Autodesk Fusion 360 part; units mm, degrees
note: some values were not read from the file. Set by a fixed rule: which face or edge a step refers to.
(part 7 of 13)
sketch "Sketch1 (3)" plane through (0, 0, 5) normal (0, 0, 1) x (-1, 0, 0)
  arc A0 (-3.482098, 1.419763) -> (-3.725467, 0.511498) centre (0, 0) ccw
  line L0 (-3.725467, 0.511498) -> (-4.55596, 0.625523)
  line L1 (-4.55596, 0.625523) -> (-4.55639, 0.625578)
  spline S0 degree 5 poles (-4.55639, 0.625578) (-4.556439, 0.625584) (-4.556519, 0.625594) (-4.556664, 0.625612) (-4.556887, 0.625638) (-4.557214, 0.625675) (-4.557589, 0.625717) (-4.558012, 0.625763) (-4.558483, 0.625812) (-4.559001, 0.625865) (-4.559566, 0.625921) (-4.560177, 0.62598) (-4.560835, 0.62604) (-4.561539, 0.626103) (-4.562289, 0.626167) (-4.563084, 0.626233) (-4.563925, 0.626299) (-4.564811, 0.626366) (-4.565742, 0.626434) (-4.566718, 0.626502) (-4.567738, 0.62657) (-4.568802, 0.626637) (-4.569909, 0.626704) (-4.571061, 0.626769) (-4.572255, 0.626834) (-4.573493, 0.626896) (-4.574774, 0.626957) (-4.576097, 0.627016) (-4.577463, 0.627072) (-4.578871, 0.627126) (-4.580321, 0.627176) (-4.581812, 0.627224) (-4.583345, 0.627268) (-4.584919, 0.627308) (-4.586534, 0.627345) (-4.58819, 0.627377) (-4.589886, 0.627405) (-4.591623, 0.627428) (-4.5934, 0.627446) (-4.595217, 0.627459) (-4.597073, 0.627467) (-4.598968, 0.627469) (-4.600903, 0.627465) (-4.602877, 0.627456) (-4.60489, 0.627439) (-4.606941, 0.627417) (-4.60903, 0.627387) (-4.611158, 0.627351) (-4.613323, 0.627308) (-4.615527, 0.627257) (-4.617767, 0.627198) (-4.620045, 0.627132) (-4.62236, 0.627058) (-4.624712, 0.626975) (-4.6271, 0.626884) (-4.629525, 0.626785) (-4.631986, 0.626676) (-4.634484, 0.626559) (-4.637017, 0.626432) (-4.639585, 0.626296) (-4.642189, 0.626151) (-4.644828, 0.625996) (-4.647503, 0.62583) (-4.650212, 0.625655) (-4.652956, 0.625469) (-4.655734, 0.625273) (-4.658546, 0.625066) (-4.661393, 0.624848) (-4.664273, 0.624619) (-4.667187, 0.624379) (-4.670135, 0.624128) (-4.673116, 0.623865) (-4.67613, 0.62359) (-4.679177, 0.623304) (-4.682256, 0.623005) (-4.685368, 0.622694) (-4.688513, 0.622371) (-4.691689, 0.622035) (-4.694898, 0.621687) (-4.698138, 0.621325) (-4.70141, 0.620951) (-4.704714, 0.620563) (-4.708048, 0.620163) (-4.711414, 0.619748) (-4.714811, 0.61932) (-4.718238, 0.618879) (-4.721696, 0.618423) (-4.725184, 0.617953) (-4.728702, 0.61747) (-4.732251, 0.616971) (-4.735829, 0.616459) (-4.739437, 0.615931) (-4.743074, 0.615389) (-4.74674, 0.614832) (-4.750436, 0.61426) (-4.754161, 0.613673) (-4.757914, 0.613071) (-4.761696, 0.612453) (-4.765506, 0.611819) (-4.769345, 0.61117) (-4.773212, 0.610505) (-4.777106, 0.609824) (-4.781029, 0.609127) (-4.784979, 0.608414) (-4.788956, 0.607684) (-4.792961, 0.606938) (-4.796992, 0.606176) (-4.801051, 0.605396) (-4.805136, 0.6046) (-4.809248, 0.603787) (-4.813386, 0.602957) (-4.817551, 0.60211) (-4.821742, 0.601246) (-4.825958, 0.600364) (-4.830201, 0.599464) (-4.834469, 0.598547) (-4.838762, 0.597613) (-4.843081, 0.59666) (-4.847425, 0.59569) (-4.851793, 0.594701) (-4.856187, 0.593695) (-4.860605, 0.59267) (-4.865048, 0.591627) (-4.869515, 0.590565) (-4.874006, 0.589485) (-4.878521, 0.588386) (-4.88306, 0.587269) (-4.887623, 0.586132) (-4.892209, 0.584977) (-4.896819, 0.583802) (-4.901452, 0.582609) (-4.906108, 0.581396) (-4.910787, 0.580163) (-4.915489, 0.578912) (-4.920213, 0.577641) (-4.92496, 0.57635) (-4.929729, 0.57504) (-4.93452, 0.573709) (-4.939334, 0.572359) (-4.944169, 0.570989) (-4.949026, 0.569599) (-4.953904, 0.568189) (-4.958804, 0.566758) (-4.963725, 0.565307) (-4.968668, 0.563836) (-4.973631, 0.562344) (-4.978615, 0.560832) (-4.98362, 0.559299) (-4.988645, 0.557746) (-4.993691, 0.556171) (-4.998756, 0.554576) (-5.003842, 0.55296) (-5.008948, 0.551323) (-5.014074, 0.549664) (-5.01922, 0.547985) (-5.024384, 0.546284) (-5.029569, 0.544562) (-5.034772, 0.542818) (-5.039995, 0.541053) (-5.045236, 0.539267) (-5.050497, 0.537458) (-5.055776, 0.535628) (-5.061073, 0.533777) (-5.066389, 0.531903) (-5.071723, 0.530008) (-5.077076, 0.528091) (-5.082446, 0.526151) (-5.087834, 0.52419) (-5.093239, 0.522206) (-5.098663, 0.5202) (-5.104103, 0.518172) (-5.109561, 0.516122) (-5.115036, 0.514049) (-5.120528, 0.511953) (-5.126037, 0.509835) (-5.131563, 0.507695) (-5.137105, 0.505532) (-5.142663, 0.503346) (-5.148238, 0.501137) (-5.153829, 0.498906) (-5.159436, 0.496651) (-5.165059, 0.494374) (-5.170698, 0.492073) (-5.176352, 0.48975) (-5.182022, 0.487404) (-5.187708, 0.485034) (-5.193408, 0.482641) (-5.199124, 0.480225) (-5.204854, 0.477785) (-5.210599, 0.475322) (-5.21636, 0.472836) (-5.222134, 0.470326) (-5.227923, 0.467793) (-5.233727, 0.465236) (-5.239544, 0.462655) (-5.245376, 0.460051) (-5.251221, 0.457423) (-5.257081, 0.454771) (-5.262954, 0.452096) (-5.26884, 0.449396) (-5.27474, 0.446673) (-5.280653, 0.443925) (-5.28658, 0.441154) (-5.292519, 0.438359) (-5.298471, 0.435539) (-5.304436, 0.432696) (-5.310414, 0.429828) (-5.316404, 0.426936) (-5.322407, 0.42402) (-5.328422, 0.421079) (-5.334448, 0.418115) (-5.340487, 0.415125) (-5.346538, 0.412112) (-5.352601, 0.409074) (-5.358675, 0.406011) (-5.364761, 0.402924) (-5.370858, 0.399812) (-5.376966, 0.396676) (-5.383086, 0.393515) (-5.389216, 0.39033) (-5.395357, 0.387119) (-5.40151, 0.383884) (-5.407672, 0.380625) (-5.413846, 0.37734) (-5.420029, 0.374031) (-5.426223, 0.370696) (-5.432428, 0.367337) (-5.438642, 0.363953) (-5.444866, 0.360544) (-5.4511, 0.35711) (-5.457343, 0.353651) (-5.463597, 0.350166) (-5.469859, 0.346657) (-5.476131, 0.343123) (-5.482412, 0.339563) (-5.488702, 0.335979) (-5.495001, 0.332369) (-5.501309, 0.328733) (-5.507626, 0.325073) (-5.513951, 0.321387) (-5.520284, 0.317676) (-5.525358, 0.314687) (-5.529167, 0.312434) (-5.531709, 0.310927) (-5.53298, 0.310172) knots 0 0 0 0 0 0 0.00416667 0.00833333 0.0125 0.01666667 0.02083333 0.025 0.02916667 0.03333333 0.0375 0.04166667 0.04583333 0.05 0.05416667 0.05833333 0.0625 0.06666667 0.07083333 0.075 0.07916667 0.08333333 0.0875 0.09166667 0.09583333 0.1 0.10416667 0.10833333 0.1125 0.11666667 0.12083333 0.125 0.12916667 0.13333333 0.1375 0.14166667 0.14583333 0.15 0.15416667 0.15833333 0.1625 0.16666667 0.17083333 0.175 0.17916667 0.18333333 0.1875 0.19166667 0.19583333 0.2 0.20416667 0.20833333 0.2125 0.21666667 0.22083333 0.225 0.22916667 0.23333333 0.2375 0.24166667 0.24583333 0.25 0.25416667 0.25833333 0.2625 0.26666667 0.27083333 0.275 0.27916667 0.28333333 0.2875 0.29166667 0.29583333 0.3 0.30416667 0.30833333 0.3125 0.31666667 0.32083333 0.325 0.32916667 0.33333333 0.3375 0.34166667 0.34583333 0.35 0.35416667 0.35833333 0.3625 0.36666667 0.37083333 0.375 0.37916667 0.38333333 0.3875 0.39166667 0.39583333 0.4 0.40416667 0.40833333 0.4125 0.41666667 0.42083333 0.425 0.42916667 0.43333333 0.4375 0.44166667 0.44583333 0.45 0.45416667 0.45833333 0.4625 0.46666667 0.47083333 0.475 0.47916667 0.48333333 0.4875 0.49166667 0.49583333 0.5 0.50416667 0.50833333 0.5125 0.51666667 0.52083333 0.525 0.52916667 0.53333333 0.5375 0.54166667 0.54583333 0.55 0.55416667 0.55833333 0.5625 0.56666667 0.57083333 0.575 0.57916667 0.58333333 0.5875 0.59166667 0.59583333 0.6 0.60416667 0.60833333 0.6125 0.61666667 0.62083333 0.625 0.62916667 0.63333333 0.6375 0.64166667 0.64583333 0.65 0.65416667 0.65833333 0.6625 0.66666667 0.67083333 0.675 0.67916667 0.68333333 0.6875 0.69166667 0.69583333 0.7 0.70416667 0.70833333 0.7125 0.71666667 0.72083333 0.725 0.72916667 0.73333333 0.7375 0.74166667 0.74583333 0.75 0.75416667 0.75833333 0.7625 0.76666667 0.77083333 0.775 0.77916667 0.78333333 0.7875 0.79166667 0.79583333 0.8 0.80416667 0.80833333 0.8125 0.81666667 0.82083333 0.825 0.82916667 0.83333333 0.8375 0.84166667 0.84583333 0.85 0.85416667 0.85833333 0.8625 0.86666667 0.87083333 0.875 0.87916667 0.88333333 0.8875 0.89166667 0.89583333 0.9 0.90416667 0.90833333 0.9125 0.91666667 0.92083333 0.925 0.92916667 0.93333333 0.9375 0.94166667 0.94583333 0.95 0.95416667 0.95833333 0.9625 0.96666667 0.97083333 0.975 0.97916667 0.98333333 0.9875 0.99166667 0.99583333 1 1 1 1 1 1
  arc A1 (-5.53298, 0.310172) -> (-5.53298, -0.310172) centre (0, 0) ccw
  spline S1 degree 5 poles (-5.53298, -0.310172) (-5.531709, -0.310927) (-5.529167, -0.312434) (-5.525358, -0.314687) (-5.520284, -0.317676) (-5.513951, -0.321387) (-5.507626, -0.325073) (-5.501309, -0.328733) (-5.495001, -0.332369) (-5.488702, -0.335979) (-5.482412, -0.339563) (-5.476131, -0.343123) (-5.469859, -0.346657) (-5.463597, -0.350166) (-5.457343, -0.353651) (-5.4511, -0.35711) (-5.444866, -0.360544) (-5.438642, -0.363953) (-5.432428, -0.367337) (-5.426223, -0.370696) (-5.420029, -0.374031) (-5.413846, -0.37734) (-5.407672, -0.380625) (-5.40151, -0.383884) (-5.395357, -0.387119) (-5.389216, -0.39033) (-5.383086, -0.393515) (-5.376966, -0.396676) (-5.370858, -0.399812) (-5.364761, -0.402924) (-5.358675, -0.406011) (-5.352601, -0.409074) (-5.346538, -0.412112) (-5.340487, -0.415125) (-5.334448, -0.418115) (-5.328422, -0.421079) (-5.322407, -0.42402) (-5.316404, -0.426936) (-5.310414, -0.429828) (-5.304436, -0.432696) (-5.298471, -0.435539) (-5.292519, -0.438359) (-5.28658, -0.441154) (-5.280653, -0.443925) (-5.27474, -0.446673) (-5.26884, -0.449396) (-5.262954, -0.452096) (-5.257081, -0.454771) (-5.251221, -0.457423) (-5.245376, -0.460051) (-5.239544, -0.462655) (-5.233727, -0.465236) (-5.227923, -0.467793) (-5.222134, -0.470326) (-5.21636, -0.472836) (-5.210599, -0.475322) (-5.204854, -0.477785) (-5.199124, -0.480225) (-5.193408, -0.482641) (-5.187708, -0.485034) (-5.182022, -0.487404) (-5.176352, -0.48975) (-5.170698, -0.492073) (-5.165059, -0.494374) (-5.159436, -0.496651) (-5.153829, -0.498906) (-5.148238, -0.501137) (-5.142663, -0.503346) (-5.137105, -0.505532) (-5.131563, -0.507695) (-5.126037, -0.509835) (-5.120528, -0.511953) (-5.115036, -0.514049) (-5.109561, -0.516122) (-5.104103, -0.518172) (-5.098663, -0.5202) (-5.093239, -0.522206) (-5.087834, -0.52419) (-5.082446, -0.526151) (-5.077076, -0.528091) (-5.071723, -0.530008) (-5.066389, -0.531903) (-5.061073, -0.533777) (-5.055776, -0.535628) (-5.050497, -0.537458) (-5.045236, -0.539267) (-5.039995, -0.541053) (-5.034772, -0.542818) (-5.029569, -0.544562) (-5.024384, -0.546284) (-5.01922, -0.547985) (-5.014074, -0.549664) (-5.008948, -0.551323) (-5.003842, -0.55296) (-4.998756, -0.554576) (-4.993691, -0.556171) (-4.988645, -0.557746) (-4.98362, -0.559299) (-4.978615, -0.560832) (-4.973631, -0.562344) (-4.968668, -0.563836) (-4.963725, -0.565307) (-4.958804, -0.566758) (-4.953904, -0.568189) (-4.949026, -0.569599) (-4.944169, -0.570989) (-4.939334, -0.572359) (-4.93452, -0.573709) (-4.929729, -0.57504) (-4.92496, -0.57635) (-4.920213, -0.577641) (-4.915489, -0.578912) (-4.910787, -0.580163) (-4.906108, -0.581396) (-4.901452, -0.582609) (-4.896819, -0.583802) (-4.892209, -0.584977) (-4.887623, -0.586132) (-4.88306, -0.587269) (-4.878521, -0.588386) (-4.874006, -0.589485) (-4.869515, -0.590565) (-4.865048, -0.591627) (-4.860605, -0.59267) (-4.856187, -0.593695) (-4.851793, -0.594701) (-4.847425, -0.59569) (-4.843081, -0.59666) (-4.838762, -0.597613) (-4.834469, -0.598547) (-4.830201, -0.599464) (-4.825958, -0.600364) (-4.821742, -0.601246) (-4.817551, -0.60211) (-4.813386, -0.602957) (-4.809248, -0.603787) (-4.805136, -0.6046) (-4.801051, -0.605396) (-4.796992, -0.606176) (-4.792961, -0.606938) (-4.788956, -0.607684) (-4.784979, -0.608414) (-4.781029, -0.609127) (-4.777106, -0.609824) (-4.773212, -0.610505) (-4.769345, -0.61117) (-4.765506, -0.611819) (-4.761696, -0.612453) (-4.757914, -0.613071) (-4.754161, -0.613673) (-4.750436, -0.61426) (-4.74674, -0.614832) (-4.743074, -0.615389) (-4.739437, -0.615931) (-4.735829, -0.616459) (-4.732251, -0.616971) (-4.728702, -0.61747) (-4.725184, -0.617953) (-4.721696, -0.618423) (-4.718238, -0.618879) (-4.714811, -0.61932) (-4.711414, -0.619748) (-4.708048, -0.620163) (-4.704714, -0.620563) (-4.70141, -0.620951) (-4.698138, -0.621325) (-4.694898, -0.621687) (-4.691689, -0.622035) (-4.688513, -0.622371) (-4.685368, -0.622694) (-4.682256, -0.623005) (-4.679177, -0.623304) (-4.67613, -0.62359) (-4.673116, -0.623865) (-4.670135, -0.624128) (-4.667187, -0.624379) (-4.664273, -0.624619) (-4.661393, -0.624848) (-4.658546, -0.625066) (-4.655734, -0.625273) (-4.652956, -0.625469) (-4.650212, -0.625655) (-4.647503, -0.62583) (-4.644828, -0.625996) (-4.642189, -0.626151) (-4.639585, -0.626296) (-4.637017, -0.626432) (-4.634484, -0.626559) (-4.631986, -0.626676) (-4.629525, -0.626785) (-4.6271, -0.626884) (-4.624712, -0.626975) (-4.62236, -0.627058) (-4.620045, -0.627132) (-4.617767, -0.627198) (-4.615527, -0.627257) (-4.613323, -0.627308) (-4.611158, -0.627351) (-4.60903, -0.627387) (-4.606941, -0.627417) (-4.60489, -0.627439) (-4.602877, -0.627456) (-4.600903, -0.627465) (-4.598968, -0.627469) (-4.597073, -0.627467) (-4.595217, -0.627459) (-4.5934, -0.627446) (-4.591623, -0.627428) (-4.589886, -0.627405) (-4.58819, -0.627377) (-4.586534, -0.627345) (-4.584919, -0.627308) (-4.583345, -0.627268) (-4.581812, -0.627224) (-4.580321, -0.627176) (-4.578871, -0.627126) (-4.577463, -0.627072) (-4.576097, -0.627016) (-4.574774, -0.626957) (-4.573493, -0.626896) (-4.572255, -0.626834) (-4.571061, -0.626769) (-4.569909, -0.626704) (-4.568802, -0.626637) (-4.567738, -0.62657) (-4.566718, -0.626502) (-4.565742, -0.626434) (-4.564811, -0.626366) (-4.563925, -0.626299) (-4.563084, -0.626233) (-4.562289, -0.626167) (-4.561539, -0.626103) (-4.560835, -0.62604) (-4.560177, -0.62598) (-4.559566, -0.625921) (-4.559001, -0.625865) (-4.558483, -0.625812) (-4.558012, -0.625763) (-4.557589, -0.625717) (-4.557214, -0.625675) (-4.556887, -0.625638) (-4.556664, -0.625612) (-4.556519, -0.625594) (-4.556439, -0.625584) (-4.55639, -0.625578) knots -1 -1 -1 -1 -1 -1 -0.99583333 -0.99166667 -0.9875 -0.98333333 -0.97916667 -0.975 -0.97083333 -0.96666667 -0.9625 -0.95833333 -0.95416667 -0.95 -0.94583333 -0.94166667 -0.9375 -0.93333333 -0.92916667 -0.925 -0.92083333 -0.91666667 -0.9125 -0.90833333 -0.90416667 -0.9 -0.89583333 -0.89166667 -0.8875 -0.88333333 -0.87916667 -0.875 -0.87083333 -0.86666667 -0.8625 -0.85833333 -0.85416667 -0.85 -0.84583333 -0.84166667 -0.8375 -0.83333333 -0.82916667 -0.825 -0.82083333 -0.81666667 -0.8125 -0.80833333 -0.80416667 -0.8 -0.79583333 -0.79166667 -0.7875 -0.78333333 -0.77916667 -0.775 -0.77083333 -0.76666667 -0.7625 -0.75833333 -0.75416667 -0.75 -0.74583333 -0.74166667 -0.7375 -0.73333333 -0.72916667 -0.725 -0.72083333 -0.71666667 -0.7125 -0.70833333 -0.70416667 -0.7 -0.69583333 -0.69166667 -0.6875 -0.68333333 -0.67916667 -0.675 -0.67083333 -0.66666667 -0.6625 -0.65833333 -0.65416667 -0.65 -0.64583333 -0.64166667 -0.6375 -0.63333333 -0.62916667 -0.625 -0.62083333 -0.61666667 -0.6125 -0.60833333 -0.60416667 -0.6 -0.59583333 -0.59166667 -0.5875 -0.58333333 -0.57916667 -0.575 -0.57083333 -0.56666667 -0.5625 -0.55833333 -0.55416667 -0.55 -0.54583333 -0.54166667 -0.5375 -0.53333333 -0.52916667 -0.525 -0.52083333 -0.51666667 -0.5125 -0.50833333 -0.50416667 -0.5 -0.49583333 -0.49166667 -0.4875 -0.48333333 -0.47916667 -0.475 -0.47083333 -0.46666667 -0.4625 -0.45833333 -0.45416667 -0.45 -0.44583333 -0.44166667 -0.4375 -0.43333333 -0.42916667 -0.425 -0.42083333 -0.41666667 -0.4125 -0.40833333 -0.40416667 -0.4 -0.39583333 -0.39166667 -0.3875 -0.38333333 -0.37916667 -0.375 -0.37083333 -0.36666667 -0.3625 -0.35833333 -0.35416667 -0.35 -0.34583333 -0.34166667 -0.3375 -0.33333333 -0.32916667 -0.325 -0.32083333 -0.31666667 -0.3125 -0.30833333 -0.30416667 -0.3 -0.29583333 -0.29166667 -0.2875 -0.28333333 -0.27916667 -0.275 -0.27083333 -0.26666667 -0.2625 -0.25833333 -0.25416667 -0.25 -0.24583333 -0.24166667 -0.2375 -0.23333333 -0.22916667 -0.225 -0.22083333 -0.21666667 -0.2125 -0.20833333 -0.20416667 -0.2 -0.19583333 -0.19166667 -0.1875 -0.18333333 -0.17916667 -0.175 -0.17083333 -0.16666667 -0.1625 -0.15833333 -0.15416667 -0.15 -0.14583333 -0.14166667 -0.1375 -0.13333333 -0.12916667 -0.125 -0.12083333 -0.11666667 -0.1125 -0.10833333 -0.10416667 -0.1 -0.09583333 -0.09166667 -0.0875 -0.08333333 -0.07916667 -0.075 -0.07083333 -0.06666667 -0.0625 -0.05833333 -0.05416667 -0.05 -0.04583333 -0.04166667 -0.0375 -0.03333333 -0.02916667 -0.025 -0.02083333 -0.01666667 -0.0125 -0.00833333 -0.00416667 0 0 0 0 0 0
  line L2 (-4.55639, -0.625578) -> (-4.55596, -0.625523)
  line L3 (-4.55596, -0.625523) -> (-3.725467, -0.511498)
  arc A2 (-3.725467, -0.511498) -> (-3.482098, -1.419763) centre (0, 0) ccw
  line L4 (-3.482098, -1.419763) -> (-4.258339, -1.736262)
  line L5 (-4.258339, -1.736262) -> (-4.258738, -1.736429)
  spline S2 degree 5 poles (-4.258738, -1.736429) (-4.258784, -1.736448) (-4.258858, -1.736479) (-4.258993, -1.736537) (-4.259199, -1.736625) (-4.259501, -1.736756) (-4.259847, -1.736908) (-4.260236, -1.73708) (-4.260668, -1.737272) (-4.261143, -1.737485) (-4.26166, -1.737719) (-4.262219, -1.737974) (-4.262819, -1.738251) (-4.26346, -1.738549) (-4.264142, -1.738868) (-4.264863, -1.739209) (-4.265625, -1.739572) (-4.266426, -1.739956) (-4.267266, -1.740363) (-4.268145, -1.740792) (-4.269062, -1.741243) (-4.270017, -1.741717) (-4.271009, -1.742213) (-4.272039, -1.742732) (-4.273106, -1.743274) (-4.274209, -1.743839) (-4.275349, -1.744426) (-4.276524, -1.745037) (-4.277735, -1.745671) (-4.278981, -1.746329) (-4.280262, -1.74701) (-4.281577, -1.747714) (-4.282927, -1.748443) (-4.28431, -1.749195) (-4.285727, -1.749971) (-4.287178, -1.750771) (-4.288661, -1.751595) (-4.290176, -1.752443) (-4.291724, -1.753316) (-4.293304, -1.754213) (-4.294915, -1.755134) (-4.296558, -1.75608) (-4.298232, -1.757051) (-4.299936, -1.758046) (-4.301671, -1.759066) (-4.303436, -1.760112) (-4.305231, -1.761182) (-4.307055, -1.762277) (-4.308909, -1.763397) (-4.310792, -1.764543) (-4.312703, -1.765714) (-4.314642, -1.76691) (-4.31661, -1.768132) (-4.318606, -1.76938) (-4.320629, -1.770653) (-4.322679, -1.771951) (-4.324756, -1.773276) (-4.32686, -1.774626) (-4.32899, -1.776002) (-4.331147, -1.777404) (-4.333329, -1.778832) (-4.335537, -1.780286) (-4.337771, -1.781766) (-4.340029, -1.783273) (-4.342312, -1.784806) (-4.34462, -1.786365) (-4.346953, -1.78795) (-4.349309, -1.789562) (-4.351689, -1.7912) (-4.354093, -1.792865) (-4.35652, -1.794557) (-4.358969, -1.796275) (-4.361442, -1.79802) (-4.363938, -1.799792) (-4.366455, -1.80159) (-4.368995, -1.803415) (-4.371557, -1.805267) (-4.37414, -1.807147) (-4.376744, -1.809053) (-4.37937, -1.810986) (-4.382016, -1.812946) (-4.384683, -1.814933) (-4.387371, -1.816948) (-4.390078, -1.818989) (-4.392806, -1.821058) (-4.395553, -1.823154) (-4.39832, -1.825278) (-4.401106, -1.827429) (-4.403911, -1.829607) (-4.406735, -1.831812) (-4.409577, -1.834046) (-4.412438, -1.836306) (-4.415317, -1.838594) (-4.418214, -1.84091) (-4.421128, -1.843253) (-4.42406, -1.845624) (-4.42701, -1.848022) (-4.429976, -1.850448) (-4.432959, -1.852902) (-4.435959, -1.855384) (-4.438975, -1.857893) (-4.442007, -1.86043) (-4.445056, -1.862995) (-4.44812, -1.865588) (-4.4512, -1.868208) (-4.454295, -1.870856) (-4.457405, -1.873533) (-4.46053, -1.876237) (-4.46367, -1.878969) (-4.466825, -1.881729) (-4.469994, -1.884517) (-4.473177, -1.887333) (-4.476374, -1.890177) (-4.479584, -1.893049) (-4.482809, -1.895949) (-4.486046, -1.898877) (-4.489297, -1.901833) (-4.492561, -1.904817) (-4.495838, -1.90783) (-4.499127, -1.91087) (-4.502429, -1.913939) (-4.505743, -1.917035) (-4.509068, -1.92016) (-4.512406, -1.923313) (-4.515756, -1.926494) (-4.519116, -1.929703) (-4.522489, -1.932941) (-4.525872, -1.936206) (-4.529266, -1.9395) (-4.532671, -1.942822) (-4.536086, -1.946172) (-4.539512, -1.949551) (-4.542948, -1.952957) (-4.546394, -1.956392) (-4.54985, -1.959855) (-4.553315, -1.963346) (-4.55679, -1.966866) (-4.560275, -1.970413) (-4.563768, -1.973989) (-4.56727, -1.977593) (-4.570782, -1.981226) (-4.574301, -1.984886) (-4.577829, -1.988575) (-4.581366, -1.992292) (-4.58491, -1.996037) (-4.588463, -1.999811) (-4.592023, -2.003613) (-4.595591, -2.007442) (-4.599166, -2.0113) (-4.602749, -2.015187) (-4.606338, -2.019101) (-4.609935, -2.023044) (-4.613538, -2.027015) (-4.617148, -2.031014) (-4.620764, -2.035041) (-4.624386, -2.039097) (-4.628015, -2.04318) (-4.63165, -2.047292) (-4.63529, -2.051432) (-4.638936, -2.0556) (-4.642588, -2.059796) (-4.646244, -2.06402) (-4.649906, -2.068272) (-4.653573, -2.072553) (-4.657245, -2.076861) (-4.660922, -2.081198) (-4.664603, -2.085562) (-4.668288, -2.089955) (-4.671978, -2.094376) (-4.675672, -2.098825) (-4.679369, -2.103301) (-4.683071, -2.107806) (-4.686776, -2.112339) (-4.690484, -2.116899) (-4.694196, -2.121488) (-4.697911, -2.126105) (-4.701629, -2.130749) (-4.70535, -2.135421) (-4.709074, -2.140122) (-4.7128, -2.14485) (-4.716528, -2.149606) (-4.720259, -2.154389) (-4.723993, -2.159201) (-4.727728, -2.16404) (-4.731465, -2.168907) (-4.735203, -2.173802) (-4.738944, -2.178725) (-4.742685, -2.183675) (-4.746428, -2.188653) (-4.750173, -2.193659) (-4.753918, -2.198692) (-4.757664, -2.203753) (-4.761411, -2.208841) (-4.765158, -2.213957) (-4.768906, -2.219101) (-4.772654, -2.224272) (-4.776403, -2.229471) (-4.780151, -2.234697) (-4.783899, -2.239951) (-4.787648, -2.245232) (-4.791395, -2.25054) (-4.795143, -2.255876) (-4.798889, -2.261239) (-4.802635, -2.26663) (-4.80638, -2.272048) (-4.810125, -2.277493) (-4.813867, -2.282965) (-4.817609, -2.288465) (-4.821349, -2.293991) (-4.825088, -2.299545) (-4.828825, -2.305126) (-4.83256, -2.310735) (-4.836294, -2.31637) (-4.840025, -2.322032) (-4.843754, -2.327722) (-4.847481, -2.333438) (-4.851205, -2.339181) (-4.854927, -2.344951) (-4.858646, -2.350749) (-4.862363, -2.356573) (-4.866076, -2.362423) (-4.869787, -2.368301) (-4.873494, -2.374206) (-4.877198, -2.380137) (-4.880899, -2.386095) (-4.884596, -2.392079) (-4.888289, -2.39809) (-4.891978, -2.404128) (-4.895664, -2.410193) (-4.899346, -2.416284) (-4.903023, -2.422401) (-4.906697, -2.428545) (-4.910366, -2.434716) (-4.91403, -2.440912) (-4.91769, -2.447136) (-4.921345, -2.453385) (-4.924995, -2.459661) (-4.92864, -2.465963) (-4.93228, -2.472291) (-4.935915, -2.478646) (-4.939545, -2.485026) (-4.942444, -2.490152) (-4.944616, -2.494008) (-4.946064, -2.496584) (-4.946787, -2.497873) knots 0 0 0 0 0 0 0.00416667 0.00833333 0.0125 0.01666667 0.02083333 0.025 0.02916667 0.03333333 0.0375 0.04166667 0.04583333 0.05 0.05416667 0.05833333 0.0625 0.06666667 0.07083333 0.075 0.07916667 0.08333333 0.0875 0.09166667 0.09583333 0.1 0.10416667 0.10833333 0.1125 0.11666667 0.12083333 0.125 0.12916667 0.13333333 0.1375 0.14166667 0.14583333 0.15 0.15416667 0.15833333 0.1625 0.16666667 0.17083333 0.175 0.17916667 0.18333333 0.1875 0.19166667 0.19583333 0.2 0.20416667 0.20833333 0.2125 0.21666667 0.22083333 0.225 0.22916667 0.23333333 0.2375 0.24166667 0.24583333 0.25 0.25416667 0.25833333 0.2625 0.26666667 0.27083333 0.275 0.27916667 0.28333333 0.2875 0.29166667 0.29583333 0.3 0.30416667 0.30833333 0.3125 0.31666667 0.32083333 0.325 0.32916667 0.33333333 0.3375 0.34166667 0.34583333 0.35 0.35416667 0.35833333 0.3625 0.36666667 0.37083333 0.375 0.37916667 0.38333333 0.3875 0.39166667 0.39583333 0.4 0.40416667 0.40833333 0.4125 0.41666667 0.42083333 0.425 0.42916667 0.43333333 0.4375 0.44166667 0.44583333 0.45 0.45416667 0.45833333 0.4625 0.46666667 0.47083333 0.475 0.47916667 0.48333333 0.4875 0.49166667 0.49583333 0.5 0.50416667 0.50833333 0.5125 0.51666667 0.52083333 0.525 0.52916667 0.53333333 0.5375 0.54166667 0.54583333 0.55 0.55416667 0.55833333 0.5625 0.56666667 0.57083333 0.575 0.57916667 0.58333333 0.5875 0.59166667 0.59583333 0.6 0.60416667 0.60833333 0.6125 0.61666667 0.62083333 0.625 0.62916667 0.63333333 0.6375 0.64166667 0.64583333 0.65 0.65416667 0.65833333 0.6625 0.66666667 0.67083333 0.675 0.67916667 0.68333333 0.6875 0.69166667 0.69583333 0.7 0.70416667 0.70833333 0.7125 0.71666667 0.72083333 0.725 0.72916667 0.73333333 0.7375 0.74166667 0.74583333 0.75 0.75416667 0.75833333 0.7625 0.76666667 0.77083333 0.775 0.77916667 0.78333333 0.7875 0.79166667 0.79583333 0.8 0.80416667 0.80833333 0.8125 0.81666667 0.82083333 0.825 0.82916667 0.83333333 0.8375 0.84166667 0.84583333 0.85 0.85416667 0.85833333 0.8625 0.86666667 0.87083333 0.875 0.87916667 0.88333333 0.8875 0.89166667 0.89583333 0.9 0.90416667 0.90833333 0.9125 0.91666667 0.92083333 0.925 0.92916667 0.93333333 0.9375 0.94166667 0.94583333 0.95 0.95416667 0.95833333 0.9625 0.96666667 0.97083333 0.975 0.97916667 0.98333333 0.9875 0.99166667 0.99583333 1 1 1 1 1 1
  arc A3 (-4.946787, -2.497873) -> (-4.636615, -3.035107) centre (0, 0) ccw
  spline S3 degree 5 poles (-4.636615, -3.035107) (-4.635137, -3.035125) (-4.632182, -3.03516) (-4.627757, -3.035206) (-4.621868, -3.035258) (-4.614528, -3.035305) (-4.607207, -3.035334) (-4.599907, -3.035346) (-4.592626, -3.03534) (-4.585366, -3.035317) (-4.578127, -3.035277) (-4.570907, -3.035219) (-4.563708, -3.035144) (-4.55653, -3.035051) (-4.549373, -3.034942) (-4.542236, -3.034816) (-4.53512, -3.034673) (-4.528025, -3.034513) (-4.520952, -3.034337) (-4.513899, -3.034144) (-4.506868, -3.033935) (-4.499858, -3.033709) (-4.492869, -3.033467) (-4.485902, -3.033209) (-4.478957, -3.032934) (-4.472033, -3.032643) (-4.465131, -3.032337) (-4.458251, -3.032015) (-4.451393, -3.031677) (-4.444557, -3.031323) (-4.437743, -3.030953) (-4.430951, -3.030569) (-4.424182, -3.030168) (-4.417435, -3.029753) (-4.410711, -3.029322) (-4.404009, -3.028876) (-4.397329, -3.028415) (-4.390673, -3.02794) (-4.384039, -3.027449) (-4.377429, -3.026944) (-4.370841, -3.026424) (-4.364277, -3.025889) (-4.357735, -3.025341) (-4.351217, -3.024777) (-4.344723, -3.0242) (-4.338252, -3.023609) (-4.331804, -3.023003) (-4.32538, -3.022384) (-4.31898, -3.021751) (-4.312603, -3.021104) (-4.306251, -3.020443) (-4.299922, -3.019769) (-4.293618, -3.019082) (-4.287338, -3.018381) (-4.281082, -3.017668) (-4.27485, -3.016941) (-4.268643, -3.016201) (-4.262461, -3.015449) (-4.256303, -3.014683) (-4.25017, -3.013905) (-4.244061, -3.013115) (-4.237978, -3.012312) (-4.231919, -3.011497) (-4.225886, -3.01067) (-4.219877, -3.009831) (-4.213894, -3.00898) (-4.207936, -3.008117) (-4.202004, -3.007242) (-4.196097, -3.006356) (-4.190216, -3.005458) (-4.184361, -3.004549) (-4.178531, -3.003629) (-4.172727, -3.002697) (-4.166949, -3.001755) (-4.161197, -3.000802) (-4.155471, -2.999838) (-4.149772, -2.998864) (-4.144098, -2.997879) (-4.138451, -2.996883) (-4.132831, -2.995878) (-4.127237, -2.994862) (-4.12167, -2.993836) (-4.11613, -2.992801) (-4.110616, -2.991756) (-4.105129, -2.990701) (-4.09967, -2.989637) (-4.094237, -2.988563) (-4.088832, -2.98748) (-4.083453, -2.986389) (-4.078103, -2.985288) (-4.072779, -2.984178) (-4.067483, -2.98306) (-4.062215, -2.981934) (-4.056975, -2.980798) (-4.051762, -2.979655) (-4.046577, -2.978504) (-4.04142, -2.977344) (-4.036292, -2.976177) (-4.031191, -2.975002) (-4.026118, -2.97382) (-4.021074, -2.97263) (-4.016059, -2.971433) (-4.011071, -2.970229) (-4.006113, -2.969018) (-4.001183, -2.9678) (-3.996281, -2.966575) (-3.991409, -2.965344) (-3.986565, -2.964107) (-3.981751, -2.962863) (-3.976965, -2.961614) (-3.972209, -2.960358) (-3.967482, -2.959097) (-3.962785, -2.95783) (-3.958116, -2.956557) (-3.953478, -2.95528) (-3.948869, -2.953997) (-3.944289, -2.952709) (-3.93974, -2.951417) (-3.93522, -2.95012) (-3.93073, -2.948818) (-3.926271, -2.947512) (-3.921841, -2.946202) (-3.917442, -2.944888) (-3.913073, -2.94357) (-3.908734, -2.942248) (-3.904426, -2.940923) (-3.900148, -2.939595) (-3.895901, -2.938263) (-3.891685, -2.936929) (-3.887499, -2.935592) (-3.883344, -2.934252) (-3.879221, -2.932909) (-3.875128, -2.931565) (-3.871067, -2.930218) (-3.867036, -2.928869) (-3.863037, -2.927519) (-3.85907, -2.926167) (-3.855134, -2.924814) (-3.851229, -2.92346) (-3.847356, -2.922104) (-3.843515, -2.920748) (-3.839706, -2.919391) (-3.835929, -2.918034) (-3.832183, -2.916676) (-3.82847, -2.915319) (-3.824789, -2.913961) (-3.82114, -2.912604) (-3.817523, -2.911247) (-3.813939, -2.909892) (-3.810387, -2.908537) (-3.806868, -2.907183) (-3.803382, -2.905831) (-3.799928, -2.90448) (-3.796507, -2.90313) (-3.793119, -2.901783) (-3.789764, -2.900438) (-3.786442, -2.899095) (-3.783153, -2.897755) (-3.779897, -2.896418) (-3.776675, -2.895084) (-3.773486, -2.893752) (-3.77033, -2.892425) (-3.767208, -2.891101) (-3.76412, -2.88978) (-3.761065, -2.888464) (-3.758045, -2.887153) (-3.755058, -2.885845) (-3.752105, -2.884543) (-3.749186, -2.883245) (-3.746301, -2.881953) (-3.74345, -2.880666) (-3.740634, -2.879385) (-3.737852, -2.87811) (-3.735105, -2.876841) (-3.732392, -2.875578) (-3.729713, -2.874322) (-3.72707, -2.873073) (-3.724461, -2.871831) (-3.721887, -2.870596) (-3.719347, -2.869369) (-3.716843, -2.86815) (-3.714374, -2.866939) (-3.71194, -2.865736) (-3.709542, -2.864542) (-3.707178, -2.863357) (-3.70485, -2.862181) (-3.702558, -2.861015) (-3.700301, -2.859858) (-3.69808, -2.858711) (-3.695894, -2.857574) (-3.693744, -2.856448) (-3.69163, -2.855332) (-3.689552, -2.854228) (-3.68751, -2.853135) (-3.685505, -2.852053) (-3.683535, -2.850983) (-3.681601, -2.849926) (-3.679704, -2.848881) (-3.677844, -2.847849) (-3.676019, -2.846829) (-3.674232, -2.845823) (-3.672481, -2.844831) (-3.670766, -2.843853) (-3.669089, -2.842888) (-3.667448, -2.841939) (-3.665845, -2.841004) (-3.664278, -2.840084) (-3.662748, -2.83918) (-3.661256, -2.838292) (-3.659801, -2.837419) (-3.658383, -2.836563) (-3.657002, -2.835724) (-3.655659, -2.834902) (-3.654354, -2.834098) (-3.653086, -2.833311) (-3.651856, -2.832542) (-3.650663, -2.831792) (-3.649509, -2.83106) (-3.648392, -2.830348) (-3.647313, -2.829655) (-3.646272, -2.828981) (-3.64527, -2.828328) (-3.644306, -2.827696) (-3.64338, -2.827085) (-3.642492, -2.826494) (-3.641642, -2.825926) (-3.640832, -2.825379) (-3.640059, -2.824855) (-3.639326, -2.824354) (-3.638631, -2.823876) (-3.637975, -2.823421) (-3.637357, -2.82299) (-3.636779, -2.822584) (-3.63624, -2.822203) (-3.635739, -2.821846) (-3.635278, -2.821515) (-3.634856, -2.821211) (-3.634473, -2.820933) (-3.63413, -2.820682) (-3.633826, -2.820458) (-3.633561, -2.820262) (-3.633381, -2.820128) (-3.633264, -2.82004) (-3.6332, -2.819991) (-3.633161, -2.819961) knots -1 -1 -1 -1 -1 -1 -0.99583333 -0.99166667 -0.9875 -0.98333333 -0.97916667 -0.975 -0.97083333 -0.96666667 -0.9625 -0.95833333 -0.95416667 -0.95 -0.94583333 -0.94166667 -0.9375 -0.93333333 -0.92916667 -0.925 -0.92083333 -0.91666667 -0.9125 -0.90833333 -0.90416667 -0.9 -0.89583333 -0.89166667 -0.8875 -0.88333333 -0.87916667 -0.875 -0.87083333 -0.86666667 -0.8625 -0.85833333 -0.85416667 -0.85 -0.84583333 -0.84166667 -0.8375 -0.83333333 -0.82916667 -0.825 -0.82083333 -0.81666667 -0.8125 -0.80833333 -0.80416667 -0.8 -0.79583333 -0.79166667 -0.7875 -0.78333333 -0.77916667 -0.775 -0.77083333 -0.76666667 -0.7625 -0.75833333 -0.75416667 -0.75 -0.74583333 -0.74166667 -0.7375 -0.73333333 -0.72916667 -0.725 -0.72083333 -0.71666667 -0.7125 -0.70833333 -0.70416667 -0.7 -0.69583333 -0.69166667 -0.6875 -0.68333333 -0.67916667 -0.675 -0.67083333 -0.66666667 -0.6625 -0.65833333 -0.65416667 -0.65 -0.64583333 -0.64166667 -0.6375 -0.63333333 -0.62916667 -0.625 -0.62083333 -0.61666667 -0.6125 -0.60833333 -0.60416667 -0.6 -0.59583333 -0.59166667 -0.5875 -0.58333333 -0.57916667 -0.575 -0.57083333 -0.56666667 -0.5625 -0.55833333 -0.55416667 -0.55 -0.54583333 -0.54166667 -0.5375 -0.53333333 -0.52916667 -0.525 -0.52083333 -0.51666667 -0.5125 -0.50833333 -0.50416667 -0.5 -0.49583333 -0.49166667 -0.4875 -0.48333333 -0.47916667 -0.475 -0.47083333 -0.46666667 -0.4625 -0.45833333 -0.45416667 -0.45 -0.44583333 -0.44166667 -0.4375 -0.43333333 -0.42916667 -0.425 -0.42083333 -0.41666667 -0.4125 -0.40833333 -0.40416667 -0.4 -0.39583333 -0.39166667 -0.3875 -0.38333333 -0.37916667 -0.375 -0.37083333 -0.36666667 -0.3625 -0.35833333 -0.35416667 -0.35 -0.34583333 -0.34166667 -0.3375 -0.33333333 -0.32916667 -0.325 -0.32083333 -0.31666667 -0.3125 -0.30833333 -0.30416667 -0.3 -0.29583333 -0.29166667 -0.2875 -0.28333333 -0.27916667 -0.275 -0.27083333 -0.26666667 -0.2625 -0.25833333 -0.25416667 -0.25 -0.24583333 -0.24166667 -0.2375 -0.23333333 -0.22916667 -0.225 -0.22083333 -0.21666667 -0.2125 -0.20833333 -0.20416667 -0.2 -0.19583333 -0.19166667 -0.1875 -0.18333333 -0.17916667 -0.175 -0.17083333 -0.16666667 -0.1625 -0.15833333 -0.15416667 -0.15 -0.14583333 -0.14166667 -0.1375 -0.13333333 -0.12916667 -0.125 -0.12083333 -0.11666667 -0.1125 -0.10833333 -0.10416667 -0.1 -0.09583333 -0.09166667 -0.0875 -0.08333333 -0.07916667 -0.075 -0.07083333 -0.06666667 -0.0625 -0.05833333 -0.05416667 -0.05 -0.04583333 -0.04166667 -0.0375 -0.03333333 -0.02916667 -0.025 -0.02083333 -0.01666667 -0.0125 -0.00833333 -0.00416667 0 0 0 0 0 0
  line L6 (-3.633161, -2.819961) -> (-3.632816, -2.819699)
  line L7 (-3.632816, -2.819699) -> (-2.9706, -2.305703)
  arc A4 (-2.9706, -2.305703) -> (-2.305703, -2.9706) centre (0, 0) ccw
  line L8 (-2.305703, -2.9706) -> (-2.819699, -3.632816)
  line L9 (-2.819699, -3.632816) -> (-2.819961, -3.633161)
  spline S4 degree 5 poles (-2.819961, -3.633161) (-2.819991, -3.6332) (-2.82004, -3.633264) (-2.820128, -3.633381) (-2.820262, -3.633561) (-2.820458, -3.633826) (-2.820682, -3.63413) (-2.820933, -3.634473) (-2.821211, -3.634856) (-2.821515, -3.635278) (-2.821846, -3.635739) (-2.822203, -3.63624) (-2.822584, -3.636779) (-2.82299, -3.637357) (-2.823421, -3.637975) (-2.823876, -3.638631) (-2.824354, -3.639326) (-2.824855, -3.640059) (-2.825379, -3.640832) (-2.825926, -3.641642) (-2.826494, -3.642492) (-2.827085, -3.64338) (-2.827696, -3.644306) (-2.828328, -3.64527) (-2.828981, -3.646272) (-2.829655, -3.647313) (-2.830348, -3.648392) (-2.83106, -3.649509) (-2.831792, -3.650663) (-2.832542, -3.651856) (-2.833311, -3.653086) (-2.834098, -3.654354) (-2.834902, -3.655659) (-2.835724, -3.657002) (-2.836563, -3.658383) (-2.837419, -3.659801) (-2.838292, -3.661256) (-2.83918, -3.662748) (-2.840084, -3.664278) (-2.841004, -3.665845) (-2.841939, -3.667448) (-2.842888, -3.669089) (-2.843853, -3.670766) (-2.844831, -3.672481) (-2.845823, -3.674232) (-2.846829, -3.676019) (-2.847849, -3.677844) (-2.848881, -3.679704) (-2.849926, -3.681601) (-2.850983, -3.683535) (-2.852053, -3.685505) (-2.853135, -3.68751) (-2.854228, -3.689552) (-2.855332, -3.69163) (-2.856448, -3.693744) (-2.857574, -3.695894) (-2.858711, -3.69808) (-2.859858, -3.700301) (-2.861015, -3.702558) (-2.862181, -3.70485) (-2.863357, -3.707178) (-2.864542, -3.709542) (-2.865736, -3.71194) (-2.866939, -3.714374) (-2.86815, -3.716843) (-2.869369, -3.719347) (-2.870596, -3.721887) (-2.871831, -3.724461) (-2.873073, -3.72707) (-2.874322, -3.729713) (-2.875578, -3.732392) (-2.876841, -3.735105) (-2.87811, -3.737852) (-2.879385, -3.740634) (-2.880666, -3.74345) (-2.881953, -3.746301) (-2.883245, -3.749186) (-2.884543, -3.752105) (-2.885845, -3.755058) (-2.887153, -3.758045) (-2.888464, -3.761065) (-2.88978, -3.76412) (-2.891101, -3.767208) (-2.892425, -3.77033) (-2.893752, -3.773486) (-2.895084, -3.776675) (-2.896418, -3.779897) (-2.897755, -3.783153) (-2.899095, -3.786442) (-2.900438, -3.789764) (-2.901783, -3.793119) (-2.90313, -3.796507) (-2.90448, -3.799928) (-2.905831, -3.803382) (-2.907183, -3.806868) (-2.908537, -3.810387) (-2.909892, -3.813939) (-2.911247, -3.817523) (-2.912604, -3.82114) (-2.913961, -3.824789) (-2.915319, -3.82847) (-2.916676, -3.832183) (-2.918034, -3.835929) (-2.919391, -3.839706) (-2.920748, -3.843515) (-2.922104, -3.847356) (-2.92346, -3.851229) (-2.924814, -3.855134) (-2.926167, -3.85907) (-2.927519, -3.863037) (-2.928869, -3.867036) (-2.930218, -3.871067) (-2.931565, -3.875128) (-2.932909, -3.879221) (-2.934252, -3.883344) (-2.935592, -3.887499) (-2.936929, -3.891685) (-2.938263, -3.895901) (-2.939595, -3.900148) (-2.940923, -3.904426) (-2.942248, -3.908734) (-2.94357, -3.913073) (-2.944888, -3.917442) (-2.946202, -3.921841) (-2.947512, -3.926271) (-2.948818, -3.93073) (-2.95012, -3.93522) (-2.951417, -3.93974) (-2.952709, -3.944289) (-2.953997, -3.948869) (-2.95528, -3.953478) (-2.956557, -3.958116) (-2.95783, -3.962785) (-2.959097, -3.967482) (-2.960358, -3.972209) (-2.961614, -3.976965) (-2.962863, -3.981751) (-2.964107, -3.986565) (-2.965344, -3.991409) (-2.966575, -3.996281) (-2.9678, -4.001183) (-2.969018, -4.006113) (-2.970229, -4.011071) (-2.971433, -4.016059) (-2.97263, -4.021074) (-2.97382, -4.026118) (-2.975002, -4.031191) (-2.976177, -4.036292) (-2.977344, -4.04142) (-2.978504, -4.046577) (-2.979655, -4.051762) (-2.980798, -4.056975) (-2.981934, -4.062215) (-2.98306, -4.067483) (-2.984178, -4.072779) (-2.985288, -4.078103) (-2.986389, -4.083453) (-2.98748, -4.088832) (-2.988563, -4.094237) (-2.989637, -4.09967) (-2.990701, -4.105129) (-2.991756, -4.110616) (-2.992801, -4.11613) (-2.993836, -4.12167) (-2.994862, -4.127237) (-2.995878, -4.132831) (-2.996883, -4.138451) (-2.997879, -4.144098) (-2.998864, -4.149772) (-2.999838, -4.155471) (-3.000802, -4.161197) (-3.001755, -4.166949) (-3.002697, -4.172727) (-3.003629, -4.178531) (-3.004549, -4.184361) (-3.005458, -4.190216) (-3.006356, -4.196097) (-3.007242, -4.202004) (-3.008117, -4.207936) (-3.00898, -4.213894) (-3.009831, -4.219877) (-3.01067, -4.225886) (-3.011497, -4.231919) (-3.012312, -4.237978) (-3.013115, -4.244061) (-3.013905, -4.25017) (-3.014683, -4.256303) (-3.015449, -4.262461) (-3.016201, -4.268643) (-3.016941, -4.27485) (-3.017668, -4.281082) (-3.018381, -4.287338) (-3.019082, -4.293618) (-3.019769, -4.299922) (-3.020443, -4.306251) (-3.021104, -4.312603) (-3.021751, -4.31898) (-3.022384, -4.32538) (-3.023003, -4.331804) (-3.023609, -4.338252) (-3.0242, -4.344723) (-3.024777, -4.351217) (-3.025341, -4.357735) (-3.025889, -4.364277) (-3.026424, -4.370841) (-3.026944, -4.377429) (-3.027449, -4.384039) (-3.02794, -4.390673) (-3.028415, -4.397329) (-3.028876, -4.404009) (-3.029322, -4.410711) (-3.029753, -4.417435) (-3.030168, -4.424182) (-3.030569, -4.430951) (-3.030953, -4.437743) (-3.031323, -4.444557) (-3.031677, -4.451393) (-3.032015, -4.458251) (-3.032337, -4.465131) (-3.032643, -4.472033) (-3.032934, -4.478957) (-3.033209, -4.485902) (-3.033467, -4.492869) (-3.033709, -4.499858) (-3.033935, -4.506868) (-3.034144, -4.513899) (-3.034337, -4.520952) (-3.034513, -4.528025) (-3.034673, -4.53512) (-3.034816, -4.542236) (-3.034942, -4.549373) (-3.035051, -4.55653) (-3.035144, -4.563708) (-3.035219, -4.570907) (-3.035277, -4.578127) (-3.035317, -4.585366) (-3.03534, -4.592626) (-3.035346, -4.599907) (-3.035334, -4.607207) (-3.035305, -4.614528) (-3.035258, -4.621868) (-3.035206, -4.627757) (-3.03516, -4.632182) (-3.035125, -4.635137) (-3.035107, -4.636615) knots 0 0 0 0 0 0 0.00416667 0.00833333 0.0125 0.01666667 0.02083333 0.025 0.02916667 0.03333333 0.0375 0.04166667 0.04583333 0.05 0.05416667 0.05833333 0.0625 0.06666667 0.07083333 0.075 0.07916667 0.08333333 0.0875 0.09166667 0.09583333 0.1 0.10416667 0.10833333 0.1125 0.11666667 0.12083333 0.125 0.12916667 0.13333333 0.1375 0.14166667 0.14583333 0.15 0.15416667 0.15833333 0.1625 0.16666667 0.17083333 0.175 0.17916667 0.18333333 0.1875 0.19166667 0.19583333 0.2 0.20416667 0.20833333 0.2125 0.21666667 0.22083333 0.225 0.22916667 0.23333333 0.2375 0.24166667 0.24583333 0.25 0.25416667 0.25833333 0.2625 0.26666667 0.27083333 0.275 0.27916667 0.28333333 0.2875 0.29166667 0.29583333 0.3 0.30416667 0.30833333 0.3125 0.31666667 0.32083333 0.325 0.32916667 0.33333333 0.3375 0.34166667 0.34583333 0.35 0.35416667 0.35833333 0.3625 0.36666667 0.37083333 0.375 0.37916667 0.38333333 0.3875 0.39166667 0.39583333 0.4 0.40416667 0.40833333 0.4125 0.41666667 0.42083333 0.425 0.42916667 0.43333333 0.4375 0.44166667 0.44583333 0.45 0.45416667 0.45833333 0.4625 0.46666667 0.47083333 0.475 0.47916667 0.48333333 0.4875 0.49166667 0.49583333 0.5 0.50416667 0.50833333 0.5125 0.51666667 0.52083333 0.525 0.52916667 0.53333333 0.5375 0.54166667 0.54583333 0.55 0.55416667 0.55833333 0.5625 0.56666667 0.57083333 0.575 0.57916667 0.58333333 0.5875 0.59166667 0.59583333 0.6 0.60416667 0.60833333 0.6125 0.61666667 0.62083333 0.625 0.62916667 0.63333333 0.6375 0.64166667 0.64583333 0.65 0.65416667 0.65833333 0.6625 0.66666667 0.67083333 0.675 0.67916667 0.68333333 0.6875 0.69166667 0.69583333 0.7 0.70416667 0.70833333 0.7125 0.71666667 0.72083333 0.725 0.72916667 0.73333333 0.7375 0.74166667 0.74583333 0.75 0.75416667 0.75833333 0.7625 0.76666667 0.77083333 0.775 0.77916667 0.78333333 0.7875 0.79166667 0.79583333 0.8 0.80416667 0.80833333 0.8125 0.81666667 0.82083333 0.825 0.82916667 0.83333333 0.8375 0.84166667 0.84583333 0.85 0.85416667 0.85833333 0.8625 0.86666667 0.87083333 0.875 0.87916667 0.88333333 0.8875 0.89166667 0.89583333 0.9 0.90416667 0.90833333 0.9125 0.91666667 0.92083333 0.925 0.92916667 0.93333333 0.9375 0.94166667 0.94583333 0.95 0.95416667 0.95833333 0.9625 0.96666667 0.97083333 0.975 0.97916667 0.98333333 0.9875 0.99166667 0.99583333 1 1 1 1 1 1
  arc A5 (-3.035107, -4.636615) -> (-2.497873, -4.946787) centre (0, 0) ccw
  spline S5 degree 5 poles (-2.497873, -4.946787) (-2.496584, -4.946064) (-2.494008, -4.944616) (-2.490152, -4.942444) (-2.485026, -4.939545) (-2.478646, -4.935915) (-2.472291, -4.93228) (-2.465963, -4.92864) (-2.459661, -4.924995) (-2.453385, -4.921345) (-2.447136, -4.91769) (-2.440912, -4.91403) (-2.434716, -4.910366) (-2.428545, -4.906697) (-2.422401, -4.903023) (-2.416284, -4.899346) (-2.410193, -4.895664) (-2.404128, -4.891978) (-2.39809, -4.888289) (-2.392079, -4.884596) (-2.386095, -4.880899) (-2.380137, -4.877198) (-2.374206, -4.873494) (-2.368301, -4.869787) (-2.362423, -4.866076) (-2.356573, -4.862363) (-2.350749, -4.858646) (-2.344951, -4.854927) (-2.339181, -4.851205) (-2.333438, -4.847481) (-2.327722, -4.843754) (-2.322032, -4.840025) (-2.31637, -4.836294) (-2.310735, -4.83256) (-2.305126, -4.828825) (-2.299545, -4.825088) (-2.293991, -4.821349) (-2.288465, -4.817609) (-2.282965, -4.813867) (-2.277493, -4.810125) (-2.272048, -4.80638) (-2.26663, -4.802635) (-2.261239, -4.798889) (-2.255876, -4.795143) (-2.25054, -4.791395) (-2.245232, -4.787648) (-2.239951, -4.783899) (-2.234697, -4.780151) (-2.229471, -4.776403) (-2.224272, -4.772654) (-2.219101, -4.768906) (-2.213957, -4.765158) (-2.208841, -4.761411) (-2.203753, -4.757664) (-2.198692, -4.753918) (-2.193659, -4.750173) (-2.188653, -4.746428) (-2.183675, -4.742685) (-2.178725, -4.738944) (-2.173802, -4.735203) (-2.168907, -4.731465) (-2.16404, -4.727728) (-2.159201, -4.723993) (-2.154389, -4.720259) (-2.149606, -4.716528) (-2.14485, -4.7128) (-2.140122, -4.709074) (-2.135421, -4.70535) (-2.130749, -4.701629) (-2.126105, -4.697911) (-2.121488, -4.694196) (-2.116899, -4.690484) (-2.112339, -4.686776) (-2.107806, -4.683071) (-2.103301, -4.679369) (-2.098825, -4.675672) (-2.094376, -4.671978) (-2.089955, -4.668288) (-2.085562, -4.664603) (-2.081198, -4.660922) (-2.076861, -4.657245) (-2.072553, -4.653573) (-2.068272, -4.649906) (-2.06402, -4.646244) (-2.059796, -4.642588) (-2.0556, -4.638936) (-2.051432, -4.63529) (-2.047292, -4.63165) (-2.04318, -4.628015) (-2.039097, -4.624386) (-2.035041, -4.620764) (-2.031014, -4.617148) (-2.027015, -4.613538) (-2.023044, -4.609935) (-2.019101, -4.606338) (-2.015187, -4.602749) (-2.0113, -4.599166) (-2.007442, -4.595591) (-2.003613, -4.592023) (-1.999811, -4.588463) (-1.996037, -4.58491) (-1.992292, -4.581366) (-1.988575, -4.577829) (-1.984886, -4.574301) (-1.981226, -4.570782) (-1.977593, -4.56727) (-1.973989, -4.563768) (-1.970413, -4.560275) (-1.966866, -4.55679) (-1.963346, -4.553315) (-1.959855, -4.54985) (-1.956392, -4.546394) (-1.952957, -4.542948) (-1.949551, -4.539512) (-1.946172, -4.536086) (-1.942822, -4.532671) (-1.9395, -4.529266) (-1.936206, -4.525872) (-1.932941, -4.522489) (-1.929703, -4.519116) (-1.926494, -4.515756) (-1.923313, -4.512406) (-1.92016, -4.509068) (-1.917035, -4.505743) (-1.913939, -4.502429) (-1.91087, -4.499127) (-1.90783, -4.495838) (-1.904817, -4.492561) (-1.901833, -4.489297) (-1.898877, -4.486046) (-1.895949, -4.482809) (-1.893049, -4.479584) (-1.890177, -4.476374) (-1.887333, -4.473177) (-1.884517, -4.469994) (-1.881729, -4.466825) (-1.878969, -4.46367) (-1.876237, -4.46053) (-1.873533, -4.457405) (-1.870856, -4.454295) (-1.868208, -4.4512) (-1.865588, -4.44812) (-1.862995, -4.445056) (-1.86043, -4.442007) (-1.857893, -4.438975) (-1.855384, -4.435959) (-1.852902, -4.432959) (-1.850448, -4.429976) (-1.848022, -4.42701) (-1.845624, -4.42406) (-1.843253, -4.421128) (-1.84091, -4.418214) (-1.838594, -4.415317) (-1.836306, -4.412438) (-1.834046, -4.409577) (-1.831812, -4.406735) (-1.829607, -4.403911) (-1.827429, -4.401106) (-1.825278, -4.39832) (-1.823154, -4.395553) (-1.821058, -4.392806) (-1.818989, -4.390078) (-1.816948, -4.387371) (-1.814933, -4.384683) (-1.812946, -4.382016) (-1.810986, -4.37937) (-1.809053, -4.376744) (-1.807147, -4.37414) (-1.805267, -4.371557) (-1.803415, -4.368995) (-1.80159, -4.366455) (-1.799792, -4.363938) (-1.79802, -4.361442) (-1.796275, -4.358969) (-1.794557, -4.35652) (-1.792865, -4.354093) (-1.7912, -4.351689) (-1.789562, -4.349309) (-1.78795, -4.346953) (-1.786365, -4.34462) (-1.784806, -4.342312) (-1.783273, -4.340029) (-1.781766, -4.337771) (-1.780286, -4.335537) (-1.778832, -4.333329) (-1.777404, -4.331147) (-1.776002, -4.32899) (-1.774626, -4.32686) (-1.773276, -4.324756) (-1.771951, -4.322679) (-1.770653, -4.320629) (-1.76938, -4.318606) (-1.768132, -4.31661) (-1.76691, -4.314642) (-1.765714, -4.312703) (-1.764543, -4.310792) (-1.763397, -4.308909) (-1.762277, -4.307055) (-1.761182, -4.305231) (-1.760112, -4.303436) (-1.759066, -4.301671) (-1.758046, -4.299936) (-1.757051, -4.298232) (-1.75608, -4.296558) (-1.755134, -4.294915) (-1.754213, -4.293304) (-1.753316, -4.291724) (-1.752443, -4.290176) (-1.751595, -4.288661) (-1.750771, -4.287178) (-1.749971, -4.285727) (-1.749195, -4.28431) (-1.748443, -4.282927) (-1.747714, -4.281577) (-1.74701, -4.280262) (-1.746329, -4.278981) (-1.745671, -4.277735) (-1.745037, -4.276524) (-1.744426, -4.275349) (-1.743839, -4.274209) (-1.743274, -4.273106) (-1.742732, -4.272039) (-1.742213, -4.271009) (-1.741717, -4.270017) (-1.741243, -4.269062) (-1.740792, -4.268145) (-1.740363, -4.267266) (-1.739956, -4.266426) (-1.739572, -4.265625) (-1.739209, -4.264863) (-1.738868, -4.264142) (-1.738549, -4.26346) (-1.738251, -4.262819) (-1.737974, -4.262219) (-1.737719, -4.26166) (-1.737485, -4.261143) (-1.737272, -4.260668) (-1.73708, -4.260236) (-1.736908, -4.259847) (-1.736756, -4.259501) (-1.736625, -4.259199) (-1.736537, -4.258993) (-1.736479, -4.258858) (-1.736448, -4.258784) (-1.736429, -4.258738) knots -1 -1 -1 -1 -1 -1 -0.99583333 -0.99166667 -0.9875 -0.98333333 -0.97916667 -0.975 -0.97083333 -0.96666667 -0.9625 -0.95833333 -0.95416667 -0.95 -0.94583333 -0.94166667 -0.9375 -0.93333333 -0.92916667 -0.925 -0.92083333 -0.91666667 -0.9125 -0.90833333 -0.90416667 -0.9 -0.89583333 -0.89166667 -0.8875 -0.88333333 -0.87916667 -0.875 -0.87083333 -0.86666667 -0.8625 -0.85833333 -0.85416667 -0.85 -0.84583333 -0.84166667 -0.8375 -0.83333333 -0.82916667 -0.825 -0.82083333 -0.81666667 -0.8125 -0.80833333 -0.80416667 -0.8 -0.79583333 -0.79166667 -0.7875 -0.78333333 -0.77916667 -0.775 -0.77083333 -0.76666667 -0.7625 -0.75833333 -0.75416667 -0.75 -0.74583333 -0.74166667 -0.7375 -0.73333333 -0.72916667 -0.725 -0.72083333 -0.71666667 -0.7125 -0.70833333 -0.70416667 -0.7 -0.69583333 -0.69166667 -0.6875 -0.68333333 -0.67916667 -0.675 -0.67083333 -0.66666667 -0.6625 -0.65833333 -0.65416667 -0.65 -0.64583333 -0.64166667 -0.6375 -0.63333333 -0.62916667 -0.625 -0.62083333 -0.61666667 -0.6125 -0.60833333 -0.60416667 -0.6 -0.59583333 -0.59166667 -0.5875 -0.58333333 -0.57916667 -0.575 -0.57083333 -0.56666667 -0.5625 -0.55833333 -0.55416667 -0.55 -0.54583333 -0.54166667 -0.5375 -0.53333333 -0.52916667 -0.525 -0.52083333 -0.51666667 -0.5125 -0.50833333 -0.50416667 -0.5 -0.49583333 -0.49166667 -0.4875 -0.48333333 -0.47916667 -0.475 -0.47083333 -0.46666667 -0.4625 -0.45833333 -0.45416667 -0.45 -0.44583333 -0.44166667 -0.4375 -0.43333333 -0.42916667 -0.425 -0.42083333 -0.41666667 -0.4125 -0.40833333 -0.40416667 -0.4 -0.39583333 -0.39166667 -0.3875 -0.38333333 -0.37916667 -0.375 -0.37083333 -0.36666667 -0.3625 -0.35833333 -0.35416667 -0.35 -0.34583333 -0.34166667 -0.3375 -0.33333333 -0.32916667 -0.325 -0.32083333 -0.31666667 -0.3125 -0.30833333 -0.30416667 -0.3 -0.29583333 -0.29166667 -0.2875 -0.28333333 -0.27916667 -0.275 -0.27083333 -0.26666667 -0.2625 -0.25833333 -0.25416667 -0.25 -0.24583333 -0.24166667 -0.2375 -0.23333333 -0.22916667 -0.225 -0.22083333 -0.21666667 -0.2125 -0.20833333 -0.20416667 -0.2 -0.19583333 -0.19166667 -0.1875 -0.18333333 -0.17916667 -0.175 -0.17083333 -0.16666667 -0.1625 -0.15833333 -0.15416667 -0.15 -0.14583333 -0.14166667 -0.1375 -0.13333333 -0.12916667 -0.125 -0.12083333 -0.11666667 -0.1125 -0.10833333 -0.10416667 -0.1 -0.09583333 -0.09166667 -0.0875 -0.08333333 -0.07916667 -0.075 -0.07083333 -0.06666667 -0.0625 -0.05833333 -0.05416667 -0.05 -0.04583333 -0.04166667 -0.0375 -0.03333333 -0.02916667 -0.025 -0.02083333 -0.01666667 -0.0125 -0.00833333 -0.00416667 0 0 0 0 0 0
  line L10 (-1.736429, -4.258738) -> (-1.736262, -4.258339)
  line L11 (-1.736262, -4.258339) -> (-1.419763, -3.482098)
  arc A6 (-1.419763, -3.482098) -> (-0.511498, -3.725467) centre (0, 0) ccw
  line L12 (-0.511498, -3.725467) -> (-0.625523, -4.55596)
  line L13 (-0.625523, -4.55596) -> (-0.625578, -4.55639)